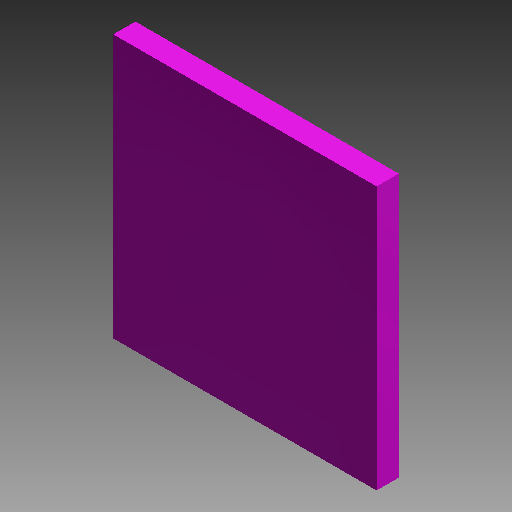
# Autodesk Inventor part: Atmega2560
Saved by Autodesk Inventor 2018.2 (Build 222227000, 227)
## iProperties
Part Number: Atmega2560
Material: Generic
Document SubType Name: Modeling
Designer: autocad
Appearance: TQFP100_140140_012, Atmega2560
Author: autocad
Autodesk Inventor part; units mm, degrees
ref_plane "YZ Plane" through (0, 0, 0) normal (1, 0, 0) x (0, 1, 0)
ref_plane "XZ Plane" through (0, 0, 0) normal (0, 1, 0) x (-1, 0, 0)
ref_plane "XY Plane" through (0, 0, 0) normal (0, 0, 1) x (1, 0, 0)
sketch "TQFP100_140140_012, Atmega2560_305" plane through (0, 0, 0) normal (0, 0, 1) x (1, 0, 0)
  line L0 (7.1374, 7.1374) -> (7.1374, -7.127)
  line L1 (7.1374, -7.127) -> (-7.127, -7.127)
  line L2 (-7.127, -7.127) -> (-7.127, 7.1374)
  line L3 (-7.127, 7.1374) -> (7.1374, 7.1374)
  constraints: 8 end point
extrude "Extrusion1" add sketch "TQFP100_140140_012, Atmega2560_305" along normal blind 1.2
body "Solid1"
